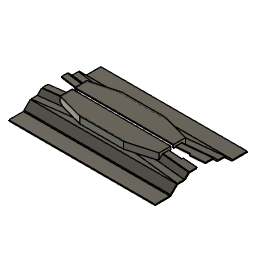
Weichenabdeckung_3Weg_beide_v2 (Autodesk Fusion 360 design; units mm, degrees)
Autodesk Fusion 360 part; units mm, degrees
sketch "Skizze1" plane through (0, 0, 0) normal (0, 0, 1) x (1, 0, 0)
  line L0 (0, 0) -> (69.6, 0)
  line L1 (69.6, 0) -> (69.6, 8)
  line L2 (51.6, 13) -> (17.6, 13)
  line L3 (0, 8.1648) -> (0, 0)
  line L4 (0, 0) -> (69.6, 0)
  line L5 (91, 2) -> (91, 32)
  line L6 (91, 32) -> (-14, 32)
  line L7 (-14, 32) -> (-14, 3.8274)
  line L8 (-14, 3.8274) -> (-0.6, 2)
  line L9 (-14, 32) -> (91, 32)
  line L10 (91, 32) -> (91, 21)
  line L11 (91, 21) -> (-14, 21)
  line L12 (-14, 21) -> (-14, 32)
  line L13 (-14, 32) -> (91, 32)
  line L14 (91, 32) -> (91, 16.0392)
  line L15 (-14, 16) -> (-14, 32)
  line L16 (-14, 32) -> (91, 32)
  line L17 (91, 32) -> (91, 11.1402)
  line L18 (-14, 11.5) -> (-14, 32)
  line L19 (-14, 32) -> (91, 32)
  line L20 (91, 32) -> (91, 7.5779)
  line L21 (-14, 8) -> (-14, 32)
  line L22 (0, 0) -> (-0.6, 0)
  line L23 (-0.6, 0) -> (70.2, 0)
  line L24 (70.2, 0) -> (70.2, 8.4561)
  line L25 (50.2418, 14) -> (18.9751, 14)
  line L26 (-14, 8) -> (-0.6, 6.2424)
  line L27 (-14, 11.5) -> (2.3256, 9.426)
  line L28 (-14, 16) -> (12.9662, 12.3492)
  line L29 (91, 16.0392) -> (56.6931, 12.208)
  line L30 (91, 11.1402) -> (68.6161, 8.896)
  line L31 (91, 7.5779) -> (70.2, 5.5847)
  line L32 (70.2, 0) -> (70.2, 1.5)
  line L33 (70.2, 1.5) -> (80.1756, 2.1976)
  line L34 (70.2, 1.5) -> (80.2, 1.5) construction
  line L35 (80.1756, 2.1976) -> (80.2367, 1.1994)
  line L36 (80.1756, 2.1976) -> (81.1795, 2.1976) construction
  line L37 (80.2367, 1.1994) -> (91, 2)
  line L38 (69.6, 0) -> (69.6, 8)
  line L39 (51.6, 13) -> (69.6, 8)
  line L40 (70.2, 8.4561) -> (50.2418, 14)
  line L41 (-0.6, 0) -> (-0.6, 8)
  line L42 (51.6, 13) -> (17.6, 13)
  line L43 (17.6, 13) -> (0, 8.1648)
  line L44 (19.0122, 14.0102) -> (-0.6, 8.6222)
  line L45 (-0.6, 8.6222) -> (-0.6, 0)
  dimension "d1" = 69.6
  dimension "d8" = 14
  dimension "d9" = 3.8274
  dimension "d13" = 2
  dimension "d14" = 32
  dimension "d15" = 105
  dimension "d16" = 11
  dimension "d17" = 16
  dimension "d18" = 20.5
  dimension "d19" = 24
  dimension "d33" = 0.6
  dimension "d34" = 70.8
  dimension "d52" = 2
  dimension "d116" = 1.5
  dimension "d117" = 10
  dimension "d118" = 4
  dimension "d119" = 86.5
  dimension "d120" = 1
  dimension "d121" = 8
  dimension "d123" = 0.6
  dimension "d125" = 8
  dimension "d126" = 18
  dimension "d127" = 34
  dimension "d129" = 0.6
  dimension "d130" = 14
  dimension "d131" = 13
  constraint horizontal L0
  constraint vertical L1
  constraint horizontal L2
  constraint vertical L3
  constraint coincident L0.start L3.end
  constraint horizontal L4
  constraint vertical L5
  constraint horizontal L6
  constraint vertical L7
  constraint coincident L3 L0.start
  constraint horizontal L9
  constraint vertical L10
  constraint horizontal L11
  constraint vertical L12
  constraint horizontal L13
  constraint vertical L14
  constraint vertical L15
  constraint horizontal L16
  constraint vertical L17
  constraint vertical L18
  constraint horizontal L19
  constraint vertical L20
  constraint vertical L21
  constraint perpendicular L3 L22
  constraint horizontal L23
  constraint vertical L24
  constraint horizontal L25
  constraint coincident L24 L31.end
  constraint perpendicular L23 L32
  constraint horizontal L34
  constraint horizontal L36
  constraint coincident L5 L20.end
  constraint coincident L5 L17.end
  constraint perpendicular L4 L38
  constraint parallel L39 L40
  constraint coincident L29.end L40
  constraint coincident L40 L30.end
  constraint perpendicular L22 L41
  constraint parallel L2 L42
  constraint parallel L43 L44
  constraint coincident L44 L25.end
  constraint coincident L28.end L44
  constraint coincident L27.end L44
  measures "d1" distance of L0.start L0.end
  measures "d8" distance of L3 L7
  measures "d9" vertical distance of L0.start L7.end
  measures "d13" distance of L0 L5.start
  measures "d14" distance of L4 L6
  measures "d15" distance of L5.end L6.end
  measures "d16" distance of L6.end L11.end
  measures "d17" distance of L6.end L15.start
  measures "d18" distance of L6.end L18.start
  measures "d19" distance of L6.end L21.start
  measures "d33" distance of L0.start L22.end
  measures "d34" distance of L22.end L23.end
  measures "d52" distance of L22.end L8.end
  measures "d116" distance of L23.end L32.end
  measures "d117" distance of L32.end L33.end
  measures "d118" angle of L33 L34
  measures "d119" angle of L35 L36
  measures "d120" distance of L33.end L35.end
  measures "d121" distance of L0.end L1.end
  measures "d123" distance of L39 L40
  measures "d125" distance of L22.end L41.end
  measures "d126" distance of L1 L2.start
  measures "d127" distance of L2.start L2.end
  measures "d129" distance of L43 L44
  measures "d130" distance of L4 L25
  measures "d131" distance of L0 L2
extrude "Extrusion1" add sketch "Skizze1" along normal blind 0.6 contours L5 L6 L7 L9 L10 L11 L12 L13 L14 L15 L16 L17 L18 L19 L20 L21 makes body 1
extrude "Extrusion2" add sketch "Skizze1" along normal blind 5.6 contours L5 L7 L11 L14 L15 L17 L18 L20 L21 L25 L28 L29 L40 L44 bodies 1
extrude "Extrusion16" add sketch "Skizze1" along normal blind 0.6 from surface at 5 separate body contours L5 L17 L20 L29 L30 L40 makes body 2
extrude "Extrusion17" add sketch "Skizze1" along normal blind 0.6 from surface at 5 separate body contours L7 L18 L21 L27 L28 L44 makes body 3
extrude "Extrusion18" add sketch "Skizze1" along normal blind 3.6 from surface at 5 separate body contours L5 L20 L24 L30 L31 L40 makes body 4
extrude "Extrusion19" add sketch "Skizze1" along normal blind 3.6 from surface at 5 separate body contours L7 L21 L26 L27 L41 L44 L45 makes body 5
extrude "Extrusion20" add sketch "Skizze1" along normal blind 0.6 from surface at 8 separate body contours L7 L8 L26 L41 L45 makes body 6
extrude "Extrusion21" add sketch "Skizze1" along normal blind 0.6 from surface at 8 separate body contours L5 L24 L31 L33 L35 L37 makes body 7
extrude "Extrusion22" add sketch "Skizze1" along normal blind 5.4 from surface at 5 separate body contours L0 L1 L2 L3 L4 L23 L38 L39 L42 L43 | L1 L2 L3 L22 L23 L24 L25 L32 L38 L39 L40 L41 L42 L43 L44 L45 makes body 8
extrude "Extrusion23" cut sketch "Skizze1" along normal blind 9.8 contours L0 L1 L2 L3 L4 L23 L38 L39 L42 L43 bodies 8
chamfer "Fase7" distance 5 angle 45 3 edges at (73.8465, 14.1236, 0) (34.6084, 14, 0) (-0.5169, 14.1746, 0) on bodies 1
chamfer "Fase8" distance 4.5 angle 45 1 edges at (38.5, 21, 5.6) on bodies 1
sketch "Skizze13" plane through (91, 0, 0) normal (1, 0, 0) x (0, 1, 0)
  line L0 (21, 1.1) -> (16.5, 5.6)
  line L1 (16.5, 5.6) -> (16.0392, 5.6)
  line L2 (16.0392, 5.6) -> (16.0392, 5)
  line L3 (16.0392, 5) -> (21.0703, 0)
  line L4 (21.0703, 0) -> (32, 0)
  line L5 (32, 0) -> (32, 0.6)
  line L6 (32, 0.6) -> (21, 0.6)
  line L7 (21, 0.6) -> (21, 1.1)
  line L8 (21, 1.1) -> (21.5, 0.6)
  line L9 (21, 0.6) -> (21, 1.1)
  constraint coincident L0.start L7.end
  constraint parallel L0 L8
  constraint coincident L6.end L7.start
extrude "Extrusion24" add sketch "Skizze13" against normal blind 105 separate body contours L6 L7 L8 L9 makes body 9
chamfer "Fase9" distance 3 angle 45 2 edges at (80.6, 6.5813, 5) (-7.3, 7.1212, 5) on bodies 4 5
chamfer "Fase10" distance 3 angle 45 2 edges at (79.808, 10.0181, 8.6) (-5.8372, 10.463, 8.6) on bodies 4 5
sketch "Skizze14" plane through (-0.6, 0, 0) normal (-1, 0, 0) x (0, -1, 0)
  line L0 (-8.6222, 5) -> (0, 5)
  line L1 (0, 10.4) -> (-8.6222, 10.4)
  line L2 (0, 5) -> (0, 8)
  line L3 (-6.2306, 8) -> (-9.2287, 5)
  line L4 (0, 5) -> (-9.2287, 5)
  line L5 (-6.2306, 8) -> (0, 8)
  line L6 (0, 5) -> (0, 10.4)
  line L7 (-8.6222, 10.4) -> (-8.6222, 5)
  dimension "d113" = 3
  constraint coincident L0.end L2.start
  constraint perpendicular L0 L2
  constraint coincident L0 L3.end
  constraint perpendicular L2 L5
  measures "d113" distance of L0.end L2.end
extrude "Extrusion25" cut sketch "Skizze14" against normal blind 105 contours L0 L2 L3 L4 L5 L6 L7 | L3 L4 L7 bodies 2 4 8
ref_plane "Arbeitsebene3" through (34.8, -1, 9.2) normal (0, -1, 0) x (1, 0, 0)
mirror "Spiegeln3" about plane through (34.8, -1, 9.2) normal (0, -1, 0) of bodies 5 7 4 1 8 9 2 6 3 makes body 10 at (37.2316, -29.4395, 0) makes body 11 at (72.1031, -14.3811, 5.6) makes body 12 at (0.4306, -14.5917, 5) makes body 13 at (84.0667, -11.2405, 6.7986) makes body 14 at (-9.5333, -11.5327, 6.9887) makes body 15 at (-5.0667, -6.0232, 8) makes body 16 at (87.3919, -5.9252, 8) makes body 17 at (39.9473, -6.6667, 10.4) makes body 18 at (56, -23.1667, 0.9333)
